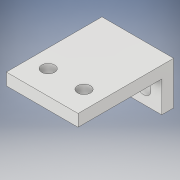
# Autodesk Inventor part: TensionerPlate4a
Saved by Autodesk Inventor 2017 (Build 210142000, 142)
## iProperties
Created: 2018-04-06
Part Number: TensionerPlate4a
Material: ABS Plastic
Document SubType Name: Modeling
Designer: User
Density: 1.06 g/cm^3
Appearance: Smooth - White
Mass: 1.89668 g
Surface Area: 15.9412 cm^2
Volume: 1.78932 cm^3
Author: User
Autodesk Inventor part; units mm, degrees
ref_plane "YZ Plane" through (0, 0, 0) normal (1, 0, 0) x (0, 1, 0)
ref_plane "XZ Plane" through (0, 0, 0) normal (0, 1, 0) x (-1, 0, 0)
ref_plane "XY Plane" through (0, 0, 0) normal (0, 0, 1) x (1, 0, 0)
sketch "Sketch1" plane through (0, 0, 0) normal (1, 0, 0) x (0, 1, 0)
  line L0 (0, 0) -> (11.43, 0)
  line L1 (11.43, 0) -> (11.43, -25.4)
  line L2 (11.43, -25.4) -> (0, -25.4)
  line L3 (0, -25.4) -> (0, 0)
  line L4 (0, 0) -> (8.255, 0)
  line L5 (8.255, 0) -> (8.255, -22.225)
  line L6 (8.255, -22.225) -> (0, -22.225)
  line L7 (0, -22.225) -> (0, 0)
  dimension "d0" = 11.43
  dimension "d1" = 25.4
  dimension "d2" = 8.255
  dimension "d3" = 22.225
  constraints: 16 end point, 4 parallel, 2 horizontal, 2 perpendicular
  measures "d0" distance of L1.end L2.end
  measures "d1" distance of L0.end L1.end
  measures "d2" distance of L5.end L6.end
  measures "d3" distance of L4.end L5.end
extrude "Extrusion1" add sketch "Sketch1" along normal blind 19.05 contours L0 L1 L2 L3 L6 L5
sketch "Sketch2" plane through (0, 11.43, 0) normal (0, 1, 0) x (1, 0, 0)
  line L0 (0, 25.4) -> (0, 0) projected
  line L1 (0, 0) -> (19.05, 0) projected
  line L2 (19.05, 25.4) -> (19.05, 0) projected
  line L3 (0, 25.4) -> (19.05, 25.4) projected
  point P0 (0, 0)
  point P1 (4.7625, 6.35)
  point P2 (14.2875, 6.35)
  dimension "d6" = 9.525
  dimension "d7" = 4.7625
  dimension "d8" = 25.4
  dimension "d31" = 19.05
  dimension "d33" = 6.35
  dimension "d34" = 6.35
  measures "d6" distance of point (14.287, 6.35) point (4.763, 6.35)
  measures "d7" distance from line of L0 point (4.763, 6.35)
  measures "d8" distance of L0.start L0.end
  measures "d31" distance of L0.end L1.end
  measures "d33" distance from line of L1 point (4.763, 6.35)
  measures "d34" distance from line of L1 point (14.287, 6.35)
hole "Hole1" at (4.7625, 11.43, -6.35) at (14.2875, 11.43, -6.35) direction (0, -1, 0) diameter 3.429 end through all
sketch "Sketch3" plane through (0, 0, -22.225) normal (0, 0, 1) x (1, 0, 0)
  line L0 (0, 0) -> (0, 8.255) projected
  line L1 (19.05, 0) -> (0, 0) projected
  line L2 (19.05, 8.255) -> (19.05, 0) projected
  line L3 (0, 8.255) -> (19.05, 8.255) projected
  point P0 (0, 0)
  point P1 (4.7625, 4.1275)
  point P2 (14.2875, 4.1275)
  dimension "d20" = 9.525
  dimension "d21" = 4.7625
  dimension "d22" = 4.1275
  dimension "d23" = 4.1275
  dimension "d32" = 19.05
  dimension "d35" = 8.255
  measures "d20" distance of point (14.287, 4.128) point (4.762, 4.128)
  measures "d21" distance from line of L2 point (14.287, 4.128)
  measures "d22" distance from line of L1 point (14.287, 4.128)
  measures "d23" distance from line of L1 point (4.762, 4.128)
  measures "d32" distance of L1.start L0.start
  measures "d35" distance of L2.start L1.start
hole "Hole2" at (4.7625, 4.1275, -22.225) at (14.2875, 4.1275, -22.225) direction (0, 0, -1) diameter 3.81 end through all
equation "\"d7\" = -0.5 * d6 + 0.5 * d31"
equation "\"d21\" = -0.5 * d20 + 0.5 * d32"
equation "\"d22\" = 0.5 * d35"
equation "\"d23\" = d22"
body "Solid1"
